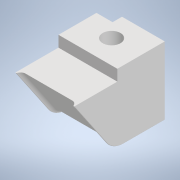
# Autodesk Inventor part: cable_slide
Saved by Autodesk Inventor 2022 (Build 260153000, 153)
## iProperties
Created: 2024-12-10
Part Number: cable_slide
Material: Типовые
Document SubType Name: Modeling
Designer: Andrey
Density: 1 g/cm^3
Appearance: По умолчанию
Author: Andrey
Autodesk Inventor part; units mm, degrees
ref_plane "YZ Plane" through (0, 0, 0) normal (1, 0, 0) x (0, 1, 0)
sketch "Эскиз1" plane through (0, 0, 0) normal (1, 0, 0) x (0, 1, 0)
  line L0 (0, 3) -> (0, 1.2702)
  line L1 (7, 3) -> (0, 3)
  line L2 (7, 3) -> (7, 0.5)
  line L3 (4.3675, 0) -> (6.5, 0)
  line L4 (0, -8.5467) -> (0, -12.5467)
  line L5 (0, -8.5467) -> (6.5, -8.5467)
  line L6 (7, -9.0467) -> (7, -12.5467)
  line L7 (0, -12.5467) -> (7, -12.5467)
  line L8 (-3, -11.0763) -> (0, -11.0763)
  line L9 (-3, 6.4737) -> (-3, -11.0763)
  line L10 (-3, 6.4737) -> (0, 6.4737)
  line L11 (0, -11.0763) -> (0, 6.4737)
  arc A0 (-11.9617, -10.4263) -> (-10.6388, -9.9263) centre (-11.9617, -8.4263) ccw
  line L12 (-12.5, -10.4263) -> (-11.9617, -10.4263)
  line L13 (-12.5, -10.4263) -> (-12.5, -5.118)
  line L14 (-3.048, -9.4263) -> (-3.048, 4.5203)
  line L15 (-9.3159, -9.4263) -> (-3.048, -9.4263)
  arc A1 (-9.3159, -9.4263) -> (-10.6388, -9.9263) centre (-9.3159, -11.4263) ccw
  line L16 (24.7127, -6.8443) -> (0, -11.2018)
  line L17 (4.1192, 0.15) -> (6.85, 0.15)
  line L18 (6.85, 0.15) -> (6.85, 2.85)
  line L19 (6.85, 2.85) -> (0.15, 2.85)
  line L20 (0.15, 2.85) -> (0.15, 1.9434)
  line L21 (6.85, -8.6967) -> (0.15, -8.6967)
  line L22 (0.15, -8.6967) -> (0.15, -12.3967)
  line L23 (0.15, -12.3967) -> (6.85, -12.3967)
  line L24 (6.85, -12.3967) -> (6.85, -8.6967)
  line L25 (0.15, 1.9434) -> (-0.15, 1.9434)
  line L26 (22.7127, -12.5467) -> (7, -12.5467)
  line L27 (6.85, -12.3967) -> (6.85, -12.5467)
  line L28 (6.85, -12.5467) -> (-9.6, -12.5467)
  line L29 (-11.5, -58.2417) -> (-11.5, -16.1467)
  line L30 (-9.6, -12.5467) -> (-9.6, -3.5467)
  line L31 (-9.6, -3.5467) -> (0, 3)
  circle A2 centre (-6.6, -5.1321) radius 3
  line L32 (6.85, 2.85) -> (6.85, 3)
  arc A3 (7, -9.0467) -> (6.5, -8.5467) centre (6.5, -9.0467) ccw
  spline S0 degree 2 poles (3.9076, 0.3039) (3.3761, 1.5505) (0.5383, 1.7687) knots -0.903693 -0.903693 -0.903693 -0.075721 -0.075721 -0.075721
  spline S1 degree 3 poles (4.3675, 0) (4.3024, 0) (4.2379, 0.0127) (4.1175, 0.0622) (4.0626, 0.0984) (3.97, 0.1898) (3.9331, 0.2441) (3.9076, 0.3039) knots 0 0 0 0 0.333468 0.333468 0.666936 0.666936 1 1 1 1
  spline S2 degree 3 poles (0, 1.2702) (0, 1.3101) (0.0048, 1.35) (0.0238, 1.4277) (0.0379, 1.4652) (0.0864, 1.5585) (0.1274, 1.6099) (0.2268, 1.694) (0.2842, 1.7259) (0.4082, 1.7659) (0.4734, 1.7737) (0.5383, 1.7687) knots 0 0 0 0 0.145255 0.145255 0.29051 0.29051 0.527006 0.527006 0.763503 0.763503 1 1 1 1
  arc A4 (6.5, 0) -> (7, 0.5) centre (6.5, 0.5) ccw
  line L33 (-9.9599, -0.2681) -> (-3.048, 4.5203)
  arc A5 (-9.9599, -0.2681) -> (-12.5, -5.118) centre (-6.6, -5.118) ccw
  circle A6 centre (6, -3.5719) radius 2.1
  circle A7 centre (25.5, 3.3533) radius 2.1
  circle A8 centre (6, 34) radius 2.1
  arc A9 (27.4853, -6.3554) -> (28.5522, -5.8) centre (27.138, -4.3858) ccw
  line L34 (27.4853, -6.3554) -> (26.9127, -6.4563)
  line L35 (26.9127, -6.4563) -> (26.9127, -0.6467)
  line L36 (26.9127, -0.6467) -> (24.7127, -0.6467)
  line L37 (24.7127, -0.6467) -> (24.7127, -6.8443)
  line L38 (24.7127, -6.8443) -> (0, -11.2018)
  line L39 (0, -11.2018) -> (0, 3)
  line L40 (0, 3) -> (14, 3)
  arc A10 (14, 3) -> (14, 29) centre (14, 16) ccw
  line L41 (14, 29) -> (0, 29)
  line L42 (0, 29) -> (0, 45.8533)
  line L43 (0, 45.8533) -> (23.2926, 28.4056)
  arc A11 (29.5, 16) -> (23.2926, 28.4056) centre (14, 16) ccw
  line L44 (29.5, 16) -> (29.5, -4.8522)
  line L45 (29.5, -4.8522) -> (28.5522, -5.8)
  line L46 (6, -12.5467) -> (6, -5.6719)
  line L47 (6, -9.1093) -> (0, -9.1093)
  line L48 (2, -7.0093) -> (2, -11.2093)
  line L49 (2, -7.0093) -> (2, -4.0093)
  line L50 (2, -4.0093) -> (0, -4.0093)
  line L51 (2, -11.2093) -> (2, -12.5467)
  point P0 (0, 0)
  point P1 (0, 1.8)
  point P2 (-8.2902, -2.6536)
  point P3 (-9.6, -5.1321)
  point P4 (2, -9.1093)
  point P5 (0, -4.0093)
  point P6 (2, -8.5467)
  dimension "d1" = 0.15
  dimension "d3" = 1.9
  dimension "d4" = 9
  dimension "d5" = 6
  dimension "d18" = 4.2
  dimension "d19" = 3
  dimension "d20" = 2
  constraints: 40 end point, 7 point on line, 6 perpendicular, 2 midpoint, 2 tangent, 1 centre point, 1 horizontal, 1 vertical, 1 vertical alignment, 10 other
  measures "d1" distance between parallel lines of L5 L21
  measures "d3" distance from line of L29 L28.end
  measures "d4" distance of L28.end L30.end
  measures "d5" diameter of A2
  measures "d18" distance of L48.start L48.end
  measures "d19" distance of L48.start L49.end
  measures "d20" distance between parallel lines of L11 L49
extrude "Выдавливание1" add sketch "Эскиз1" along normal mid plane 10.6 contours L0 L11 L4 L8 L9 L31 | L9 L8 L4 L28 L30 A1 L15 L14 L31 | L14 L15 A1 L30 A2 L31 | L50 L49 L48 L5 L11 | L4 L47 L22 L16 | A2 | L5 L48 L21 L22 L47 L4 | L16 L22 L23 L51 L7 L4 | L47 L48 L16 L22 | L22 L21 L48 L47 | L16 L48 L51 L23 L22
ref_plane "РабПлоскость1" through (-2.4, 7, -12.5467) normal (-1, 0, 0) x (0, 0, 1)
sketch "Эскиз4" plane through (-5.3, -9.6, -12.5467) normal (0, -1, 0) x (1, 0, 0)
  line L0 (0, 8.5374) -> (10.6, 8.5374) projected
  line L1 (10.6, 0) -> (10.6, 8.5374) projected
  line L2 (0, 0) -> (10.6, 0) projected
  line L3 (0, 8.5374) -> (0, 0) projected
  line L4 (5.3, 8.5374) -> (5.3, 0)
  circle A0 centre (5.3, 4.2687) radius 1.6
  point P0 (5.3, 12.5467)
  dimension "d21" = 3.2
  constraints: 3 midpoint, 2 end point, 1 centre point
  measures "d21" diameter of A0
extrude "Выдавливание4" cut sketch "Эскиз4" against normal blind 12 contours A0 L4 | L4 A0
sketch "Эскиз5" plane through (-5.3, -9.6, -12.5467) normal (0, -1, 0) x (1, 0, 0)
  circle A0 centre (5.3, 4.2687) radius 1.6 projected
  line L0 (10.6, 0) -> (0, 0) projected
  line L1 (10.6, 7.4147) -> (10.6, 0) projected
  line L2 (0, 7.4147) -> (10.6, 7.4147) projected
  line L3 (0, 0) -> (0, 7.4147) projected
  circle A1 centre (5.3, 4.2687) radius 2.75
  point P0 (5.3, 12.5467)
  dimension "d24" = 5.5
  constraints: 1 centre point, 1 coincident
  measures "d24" diameter of A1
extrude "Выдавливание5" cut sketch "Эскиз5" against normal blind 3.4 contours A1
sketch "Эскиз6" plane through (-5.3, 0, 0) normal (-1, 0, 0) x (0, 0, 1)
  line L0 (-4.0093, 2) -> (-4.0093, 0) projected
  line L1 (-4.0093, 0) -> (3, 0) projected
  line L2 (3, 0) -> (3, 14) projected
  arc A0 (29, 14) -> (3, 14) centre (16, 14) ccw projected
  line L3 (29, 14) -> (29, 0) projected
  line L4 (29, 0) -> (45.8533, 0) projected
  line L5 (45.8533, 0) -> (28.4056, 23.2926) projected
  arc A1 (28.4056, 23.2926) -> (16, 29.5) centre (16, 14) ccw projected
  line L6 (16, 29.5) -> (-4.8522, 29.5) projected
  line L7 (-4.8522, 29.5) -> (-5.8, 28.5522) projected
  arc A2 (-5.8, 28.5522) -> (-6.3554, 27.4853) centre (-4.3858, 27.138) ccw projected
  line L8 (-6.3554, 27.4853) -> (-6.4563, 26.9127) projected
  line L9 (-6.4563, 26.9127) -> (-0.6467, 26.9127) projected
  line L10 (-0.6467, 26.9127) -> (-0.6467, 24.7127) projected
  line L11 (-0.6467, 24.7127) -> (-6.8443, 24.7127) projected
  line L12 (-6.8443, 24.7127) -> (-10.8491, 2) projected
  circle A3 centre (-3.5719, 6) radius 2.1 projected
  circle A4 centre (3.3533, 25.5) radius 2.1 projected
  circle A5 centre (34, 6) radius 2.1 projected
  line L13 (-6.8443, 24.7127) -> (-10.8491, 2) projected
  line L14 (-6.8443, 24.7127) -> (-10.5467, 24.7127) projected
  line L15 (-12.5467, 22.7127) -> (-10.5467, 24.7127) projected
  line L16 (-12.5467, 22.7127) -> (-12.5467, 2) projected
  line L17 (-10.8491, 2) -> (-12.5467, -7.6277)
  line L18 (-12.5467, 2) -> (-12.5467, -9.6) projected
  line L19 (-10.8491, 2) -> (-4.0093, 2) projected
  line L20 (-12.5467, 2) -> (-10.8491, 2) projected
  point P0 (0, 0)
  constraints: 2 end point, 1 collinear, 1 point on line
ref_plane "РабПлоскость2" through (-2.4, 2, -12.5467) normal (-1, 0, 0) x (0, 0, 1)
extrude "Выдавливание6" cut sketch "Эскиз6" against normal up to surface (2.9 mm away) contours L17 L18 L20
sketch "Эскиз7" plane through (-5.3, 0, 0) normal (-1, 0, 0) x (0, 0, 1)
  line L0 (-10.8491, 2) -> (-12.5467, -7.6277) projected
  line L1 (-12.5467, -7.6277) -> (-12.5467, -9.6) projected
  line L2 (-12.5467, -9.6) -> (-5.1321, -9.6) projected
  arc A0 (-5.1321, -9.6) -> (-2.6536, -8.2902) centre (-5.1321, -6.6) ccw projected
  line L3 (-2.6536, -8.2902) -> (3, 0) projected
  line L4 (3, 0) -> (-4.0093, 0) projected
  line L5 (-4.0093, 0) -> (-4.0093, 2) projected
  line L6 (-4.0093, 2) -> (-10.8491, 2) projected
  arc A1 (-5.1321, -10.6) -> (-1.8274, -8.8537) centre (-5.1321, -6.6) ccw
  line L7 (-5.1321, -10.6) -> (-13.5467, -10.6)
  line L8 (-13.5467, -10.6) -> (-13.5467, -7.5402)
  line L9 (-13.5467, -7.5402) -> (-11.6882, 3)
  line L10 (-11.6882, 3) -> (-3.0093, 3)
  line L11 (-3.0093, 3) -> (-3.0093, 1)
  line L12 (-3.0093, 1) -> (4.8923, 1)
  line L13 (4.8923, 1) -> (-1.8274, -8.8537)
  line L14 (-4.0093, 0) -> (3, 0) projected
  line L15 (3, 0) -> (4.2104, 0)
  line L16 (-12.5467, -9.6) -> (-12.5467, 2) projected
  line L17 (-12.5467, -9.6) -> (-12.5467, -10.6)
  point P0 (0, 0)
  dimension "d29" = 1
  constraints: 18 end point, 3 point on line, 2 point on circle, 1 centre point, 1 collinear, 7 other
  measures "d29" radial gap between concentric circles of A0 A1
extrude "Выдавливание7" add sketch "Эскиз7" against normal blind 1.1 contours L2 A0 L3 L15 L13 A1 L7 L17
fillet "Сопряжение4" radius 1 3 edges at (-4.2, -10.1366, -3.2632) (-4.2, -4.4268, 1.1915) (-4.2, -10.6, -8.8394) inverted yes
fillet "Сопряжение5" radius 0.1 6 edges at (-5.3, -10.1366, -3.2632) (-5.3, -4.4268, 1.1915) (-5.3, -10.6, -8.8394) (-5.2, -10.6, -8.8394) (-5.2, -4.4268, 1.1915) (-5.2, -10.1366, -3.2632)
mirror "Зеркальное отражение1" about plane through (0, 0, 0) normal (1, 0, 0) of "Выдавливание7", "Сопряжение4", "Сопряжение5"
